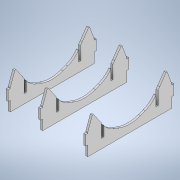
# Autodesk Inventor part: dno
Saved by Autodesk Inventor 2020 (Build 240168000, 168)
## iProperties
Created: 2022-01-10
Part Number: dno
Material: Типовые
Document SubType Name: Modeling
Designer: solidworks
Density: 1 g/cm^3
Appearance: По умолчанию
Author: solidworks
Autodesk Inventor part; units mm, degrees
ref_plane "YZ Plane" through (0, 0, 0) normal (1, 0, 0) x (0, 1, 0)
ref_plane "XZ Plane" through (0, 0, 0) normal (0, 1, 0) x (-1, 0, 0)
sketch "Эскиз1" plane through (0, 0, 0) normal (0, 1, 0) x (-1, 0, 0)
  line L0 (-8, 0) -> (-8, 332)
  line L1 (-8, 332) -> (2, 332)
  line L2 (-8, 0) -> (-178, 0) construction
  line L3 (-178, 332) -> (-187.2412, 332)
  line L4 (-168, 0) -> (-178, 0)
  line L5 (2, 332) -> (0, 332)
  line L6 (0, 332) -> (0, 0)
  line L7 (120, 332) -> (120, 0)
  line L8 (0, 0) -> (-8, 0)
  line L9 (-168, 0) -> (-186, 0)
  line L10 (-186, 0) -> (-186, 332)
  line L11 (-186, 332) -> (-187.2412, 332)
  line L12 (-178, 332) -> (-178, 0)
  line L13 (128, 0) -> (128, 332)
  line L14 (120, 0) -> (128, 0)
  line L15 (120, 332) -> (128, 332)
  point P0 (0, 0)
  point P1 (-166, 0)
  point P2 (-178, 0)
  dimension "d1" = 332
  dimension "d2" = 170
  dimension "d18" = 8
  dimension "d25" = 8
  dimension "d26" = 120
  dimension "d27" = 8
  dimension "d28" = 0
  constraints: 32 end point, 5 horizontal, 5 perpendicular, 2 vertical, 1 parallel, 1 point on line
  measures "d1" distance of L0.start L0.end
  measures "d2" distance of L0.start L2.end
  measures "d18" distance of L6.end L0.start
  measures "d25" distance of L9.end L2.end
  measures "d26" distance between parallel lines of L7 L6
  measures "d27" distance between parallel lines of L13 L7
  measures "d28" distance from line of L6 point (0, 0)
extrude "Выдавливание1" add sketch "Эскиз1" along normal blind 166
sketch "Эскиз2" plane through (-130, 0, 0) normal (-1, 0, 0) x (0, 0, 1)
  line L0 (0, 0) -> (0, 166) construction
  line L1 (332, 0) -> (332, 166) construction
  line L2 (0, 166) -> (166, 166) construction
  circle A0 centre (166, 166) radius 136 construction
  line L3 (104.8926, 43.667) -> (123.8668, 36.552)
  line L4 (227.1074, 43.667) -> (208.1332, 36.552)
  arc A1 (123.8668, 36.552) -> (208.1332, 36.552) centre (166, 148.9121) ccw
  line L5 (0, 166) -> (332, 166) construction
  line L6 (22.6502, 133.6372) -> (54.5783, 88.0179)
  line L7 (54.5783, 88.0179) -> (62.7576, 76.3313)
  line L8 (0, 83) -> (18.0836, 133.0313)
  arc A2 (62.7576, 76.3313) -> (104.8926, 43.667) centre (136.4925, 127.9371) ccw
  line L9 (22.6502, 133.6372) -> (18.0836, 133.0313)
  line L10 (166, 166) -> (166, 148.9121) construction
  line L11 (309.3498, 133.6372) -> (277.4217, 88.0179)
  line L12 (277.4217, 88.0179) -> (269.2424, 76.3313)
  line L13 (332, 83) -> (313.9164, 133.0313)
  arc A3 (227.1074, 43.667) -> (269.2424, 76.3313) centre (195.5075, 127.9371) ccw
  line L14 (309.3498, 133.6372) -> (313.9164, 133.0313)
  line L15 (332, 83) -> (332, 166)
  line L16 (332, 166) -> (0, 166)
  line L17 (0, 166) -> (0, 83)
  point P0 (19.7832, 137.7335)
  dimension "d10" = 272
  dimension "d11" = 120
  dimension "d12" = 90
  dimension "d13" = 5
  dimension "d14" = 5
  constraints: 30 end point, 6 point on circle, 6 symmetric about line, 4 tangent, 3 centre point, 3 perpendicular, 2 midpoint, 2 point on line, 1 coincident, 1 vertical, 8 other
  measures "d11" radius of A1
  measures "d12" radius of A2
  measures "d13" distance of L6.start point (19.783, 137.734)
  measures "d14" distance of L8.end point (19.783, 137.734)
ref_plane "РабПлоскость1" through (0, 0, 166) normal (0, 0, 1) x (1, 0, 0)
sketch "Эскиз4" plane through (-128, 0, 0) normal (-1, 0, 0) x (0, 0, 1)
  line L0 (0, 0) -> (0, 166) construction
  line L1 (332, 0) -> (332, 166) construction
  line L2 (0, 166) -> (166, 166) construction
  arc A0 (277.6, 88.2733) -> (213.751, 38.6585) centre (166, 166) ccw construction
  line L3 (104.8926, 43.667) -> (123.8668, 36.552)
  line L4 (227.1074, 43.667) -> (208.1332, 36.552)
  arc A1 (123.8668, 36.552) -> (208.1332, 36.552) centre (166, 148.9121) ccw
  line L5 (0, 166) -> (332, 166) construction
  line L6 (22.6502, 133.6372) -> (47.822, 97.6714)
  line L7 (0, 83) -> (18.0836, 133.0313)
  arc A2 (62.7576, 76.3313) -> (104.8926, 43.667) centre (136.4925, 127.9371) ccw
  line L8 (22.6502, 133.6372) -> (18.0836, 133.0313)
  line L9 (166, 166) -> (166, 148.9121) construction
  line L10 (309.3498, 133.6372) -> (284.178, 97.6714)
  line L11 (332, 83) -> (313.9164, 133.0313)
  line L12 (309.3498, 133.6372) -> (313.9164, 133.0313)
  arc A3 (227.1074, 43.667) -> (269.2424, 76.3313) centre (195.5075, 127.9371) ccw
  line L13 (332, 83) -> (332, 166)
  line L14 (332, 166) -> (0, 166)
  line L15 (0, 166) -> (0, 83)
  line L16 (54.4, 106.4464) -> (54.4, 143.4464) projected
  line L17 (54.4, 88.2733) -> (54.4, 36.552)
  line L18 (54.4, 36.552) -> (62.4, 36.552)
  line L19 (62.4, 36.552) -> (62.4, 76.846)
  line L20 (47.822, 97.6714) -> (54.4, 88.2733)
  line L21 (62.4, 76.846) -> (62.7576, 76.3313)
  line L22 (277.6, 88.2733) -> (277.6, 36.552)
  line L23 (277.6, 36.552) -> (269.6, 36.552)
  line L24 (269.6, 36.552) -> (269.6, 76.846)
  line L25 (269.2424, 76.3313) -> (269.6, 76.846)
  line L26 (284.178, 97.6714) -> (277.6, 88.2733)
  point P0 (0, 0)
  point P1 (54.5783, 88.0179)
  point P2 (19.7832, 137.7335)
  point P3 (277.4217, 88.0179)
  point P4 (283.0312, 96.0329)
  point P5 (48.9688, 96.0329)
  dimension "d29" = 272
  dimension "d30" = 120
  dimension "d31" = 90
  dimension "d32" = 5
  dimension "d33" = 5
  dimension "d46" = 2
  dimension "d50" = 2
  dimension "d53" = 8
  dimension "d54" = 90
  constraints: 52 end point, 11 point on circle, 11 symmetric about line, 6 tangent, 5 point on line, 4 centre point, 3 perpendicular, 2 midpoint, 2 vertical, 1 coincident, 1 horizontal, 1 other
  measures "d29" diameter of A0
  measures "d30" radius of A1
  measures "d31" radius of A2
  measures "d32" distance of L6.start point (19.783, 137.734)
  measures "d33" distance of L7.end point (19.783, 137.734)
  measures "d46" distance of L6.end point (48.969, 96.033)
  measures "d50" distance of L10.end point (283.031, 96.033)
  measures "d53" distance of L17.end L18.end
  measures "d54" angle of L19 L18
extrude "Выдавливание4" cut sketch "Эскиз4" against normal through all
sketch "Эскиз5" plane through (178, 0, 332) normal (0, 0, 1) x (1, 0, 0)
  line L0 (39.2204, 40) -> (-44.3448, 40) construction
  line L1 (39.2204, 0) -> (-44.3448, 0) construction
  line L2 (8, 0) -> (8, 83) projected
  line L3 (8, 40) -> (0, 40)
  line L4 (0, 40) -> (0, 80)
  line L5 (0, 80) -> (8, 80)
  line L6 (8, 80) -> (8, 40)
  line L7 (-44.3448, 40) -> (-315.6542, 40) construction
  line L8 (-170, 36.552) -> (-170, 43.667) projected
  line L9 (-178, 133.6372) -> (-178, 97.6714) projected
  line L10 (-170, 40.1095) -> (-178, 40.1095)
  line L11 (-178, 40.1095) -> (-178, 80.1095)
  line L12 (-178, 80.1095) -> (-170, 80.1095)
  line L13 (-170, 80.1095) -> (-170, 40.1095)
  line L14 (-306, 36.552) -> (-306, 43.667) projected
  line L15 (-298, 0) -> (-298, 83) projected
  line L16 (-306, 40.1095) -> (-298, 40.1095)
  line L17 (-298, 40.1095) -> (-298, 80.1095)
  line L18 (-298, 80.1095) -> (-306, 80.1095)
  line L19 (-306, 80.1095) -> (-306, 40.1095)
  point P0 (-178, 0)
  point P1 (-178, 76.3313)
  point P2 (-178, 76.3313)
  dimension "d36" = 40
  dimension "d37" = 8
  dimension "d38" = 40
  dimension "d39" = 40
  constraints: 30 end point, 6 horizontal, 6 parallel, 5 point on line, 3 perpendicular, 2 midpoint
  measures "d36" distance between parallel lines of L0 L1
  measures "d37" distance of L4.end L5.end
  measures "d38" distance of L3.end L4.end
  measures "d39" distance of L10.end L11.end
extrude "Выдавливание5" add sketch "Эскиз5" along normal blind 8
mirror "Зеркальное отражение2" about plane through (0, 0, 166) normal (0, 0, 1) of "Выдавливание5"
equation "\"d14\" = d13"
equation "\"d33\" = d32"
equation "\"d46\" = d45"
equation "\"d50\" = d49"
equation "\"d45\" = d43"
equation "\"d49\" = d43"
equation "\"d43\" = 2"
